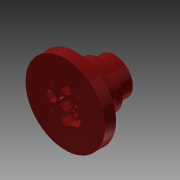
# Autodesk Inventor part: stand_coupler1
Saved by Autodesk Inventor 2013 (Build 170138000, 138)
## iProperties
Created: 2014-10-25
Part Number: stand_coupler1
Material: ABS Plastic
Document SubType Name: Modeling
Designer: Masta
Density: 1 g/cm^3
Author: Masta
Autodesk Inventor part; units mm, degrees
ref_plane "YZ Plane" through (0, 0, 0) normal (1, 0, 0) x (0, 1, 0)
ref_plane "XZ Plane" through (0, 0, 0) normal (0, 1, 0) x (-1, 0, 0)
ref_plane "XY Plane" through (0, 0, 0) normal (0, 0, 1) x (1, 0, 0)
sketch "Sketch1" plane through (0, 0, 0) normal (1, 0, 0) x (0, 1, 0)
  line L0 (0, 0) -> (0, 32.5)
  line L1 (0, 0) -> (40.5, 0)
  line L2 (23, 18.5) -> (28.5, 18.5)
  line L3 (28.5, 18.5) -> (28.5, 14.75)
  line L4 (28.5, 14.75) -> (40.5, 14.75)
  line L5 (40.5, 14.75) -> (40.5, 0)
  line L6 (0, 32.5) -> (9, 32.5)
  line L7 (9, 32.5) -> (9, 22.25)
  line L8 (9, 22.25) -> (12, 22.25)
  line L9 (12, 22.25) -> (23, 18.5)
  dimension "d0" = 32.5
  dimension "d1" = 12
  dimension "d2" = 14.75
  dimension "d4" = 18.5
  dimension "d5" = 5.5
  dimension "d6" = 14
  dimension "d7" = 3
  dimension "d8" = 9
  dimension "d9" = 22.25
  constraints: 21 end point, 6 perpendicular, 2 parallel, 1 vertical
  measures "d0" distance of L0.start L0.end
  measures "d1" distance of L3.end L4.end
  measures "d2" distance of L4.end L1.end
  measures "d4" distance between parallel lines of L1 L2
  measures "d5" distance of L2.start L2.end
  measures "d6" distance from line of L2.start L7
  measures "d7" distance of L7.end L8.end
  measures "d8" distance of L0.end L6.end
  measures "d9" distance between parallel lines of L1 L8
revolve "Revolution1" add sketch "Sketch1" angle 360 about axis through (0, 0, 0) along (0, 1, 0)
sketch "Sketch2" plane through (0, 40.5, 0) normal (0, 1, 0) x (1, 0, 0)
  circle A0 centre (0, 0) radius 14.75 projected
  line L0 (0, 0) -> (11, 0) construction
  dimension "d11" = 11
  constraints: 2 end point, 1 coincident, 1 horizontal
  measures "d11" distance of L0.start L0.end
hole "Hole1" at (11, 40.5, 0) direction (0, -1, 0) diameter 4.5 end through all
hole "Hole2" at (0, 40.5, 0) direction (0, -1, 0) diameter 10 end through all
sketch "Sketch3" plane through (0, 0, 0) normal (0, -1, 0) x (1, 0, 0)
  line L0 (15.3301, 0) -> (13.1651, -3.75)
  line L1 (13.1651, -3.75) -> (8.8349, -3.75)
  line L2 (8.8349, -3.75) -> (6.6699, 0)
  line L3 (6.6699, 0) -> (8.8349, 3.75)
  line L4 (8.8349, 3.75) -> (13.1651, 3.75)
  line L5 (13.1651, 3.75) -> (15.3301, 0)
  circle A0 centre (11, 0) radius 2.25 projected
  circle A1 centre (0, 0) radius 32.5 projected
  line L6 (11, 0) -> (0, 0) construction
  line L7 (0, 0) -> (10.253, -10.253) construction
  point P0 (11, 0)
  dimension "d31" = 7.5
  dimension "d37" = 14.5
  dimension "d38" = 45
  constraints: 16 end point, 2 coincident, 1 parallel, 13 other
  measures "d31" distance between parallel lines of L1 L4
  measures "d37" distance of L6.end L7.end
  measures "d38" angle of L6 L7
extrude "Extrusion1" cut sketch "Sketch3" against normal blind 8 contours L0 L1 L2 L3 L4 L5 | A0
hole "Hole3" at (10.253, 0, -10.253) direction (0, 1, 0) diameter 2 depth 15 tip angle 118
pattern_circular "Circular Pattern2" count 4 over 360 about axis through (0, -10, 0) along (0, 1, 0) of "Extrusion1", "Hole1", "Hole3"
sketch "Sketch4" plane through (0, 0, 0) normal (0, -1, 0) x (1, 0, 0)
  line L0 (0, -6.6699) -> (3.75, -8.8349) projected
  line L1 (3.75, -8.8349) -> (3.75, -13.1651) projected
  circle A0 centre (10.253, -10.253) radius 1 projected
  line L2 (13.1651, -3.75) -> (8.8349, -3.75) projected
  line L3 (8.8349, -3.75) -> (6.6699, 0) projected
  line L4 (8.8349, 3.75) -> (13.1651, 3.75) projected
  circle A1 centre (0, 0) radius 32.5 projected
  line L5 (0, -6.6699) -> (0, 0)
  line L6 (0, 0) -> (6.6699, 0)
  line L7 (3.75, -13.1651) -> (10.5296, -11.214)
  line L8 (13.1651, -3.75) -> (11.214, -10.5296)
  constraints: 8 end point, 2 perpendicular, 2 point on circle, 2 tangent
extrude "Extrusion2" cut sketch "Sketch4" against normal up to surface (8 mm away) contours L5 L6 L3 L2 L8 A0 L7 L1 L0
body "Solid1"
